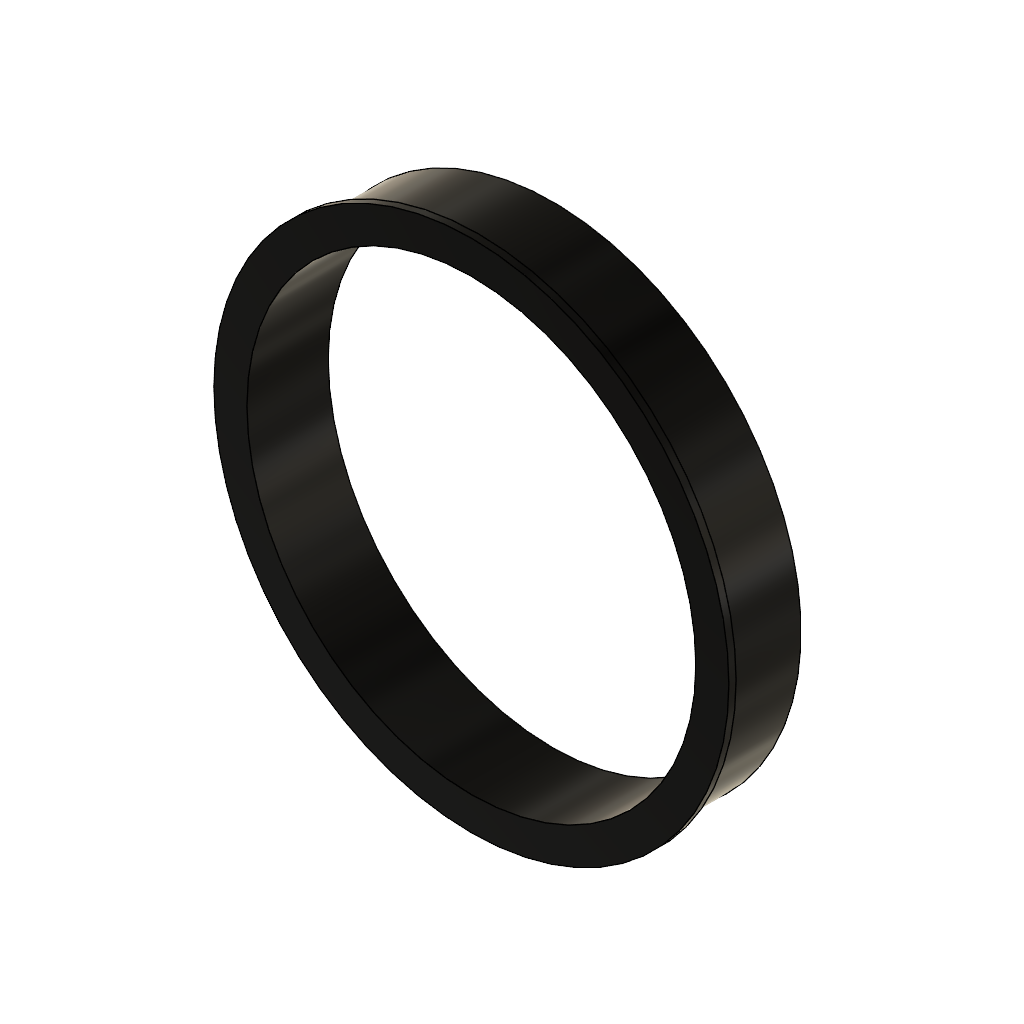
Rick Workshop cache difusant led (Autodesk Fusion 360 design; units mm, degrees)
Autodesk Fusion 360 part; units mm, degrees
(part 1 of 2)
sketch "Esquisse261" plane through (0, 0, 0) normal (0, 1, 0) x (1, 0, 0)
  spline S0 degree 5 poles (130.1631, -52) (130.1652, -52.1909) (130.1668, -52.5728) (130.1613, -53.1457) (130.1382, -53.9093) (130.0834, -54.8626) (130.0031, -55.814) (129.8983, -56.7629) (129.77, -57.7086) (129.6195, -58.6508) (129.4486, -59.5891) (129.2587, -60.5234) (129.0517, -61.4536) (128.8294, -62.3797) (128.5934, -63.3018) (128.3453, -64.2202) (128.0865, -65.1352) (127.8182, -66.0469) (127.5414, -66.9556) (127.2566, -67.8616) (126.9641, -68.7649) (126.6638, -69.6656) (126.3553, -70.5636) (126.0379, -71.4586) (125.7105, -72.3502) (125.372, -73.238) (125.0207, -74.1211) (124.6551, -74.9988) (124.2736, -75.8699) (123.8744, -76.7335) (123.4561, -77.5881) (123.0173, -78.4325) (122.5566, -79.2654) (122.0732, -80.0853) (121.5664, -80.891) (121.0359, -81.6814) (120.482, -82.4553) (119.9049, -83.212) (119.3056, -83.951) (118.685, -84.672) (118.0445, -85.3749) (117.3859, -86.0604) (116.7109, -86.7289) (116.0215, -87.3814) (115.3196, -88.0193) (114.6071, -88.6438) (113.8861, -89.2567) (113.1582, -89.8597) (112.4253, -90.4544) (111.6886, -91.0426) (110.9496, -91.6259) (110.2091, -92.2056) (109.4678, -92.7829) (108.7262, -93.3586) (107.9842, -93.9332) (107.2416, -94.5069) (106.4979, -95.0792) (105.7522, -95.6496) (105.0035, -96.2171) (104.2507, -96.7802) (103.4926, -97.3374) (102.7276, -97.8865) (101.9545, -98.4256) (101.1721, -98.9523) (100.3792, -99.4643) (99.5749, -99.9593) (98.7586, -100.4349) (97.9298, -100.8889) (97.0882, -101.3195) (96.234, -101.7248) (95.3676, -102.1035) (94.4896, -102.4546) (93.6008, -102.7773) (92.7022, -103.0714) (91.7948, -103.337) (90.8799, -103.5747) (89.9586, -103.7854) (89.032, -103.9704) (88.1014, -104.1309) (87.1676, -104.2689) (86.2317, -104.3859) (85.2943, -104.484) (84.3561, -104.565) (83.4176, -104.6306) (82.4793, -104.6826) (81.5414, -104.7223) (80.604, -104.751) (79.6674, -104.7697) (78.7314, -104.7791) (77.7963, -104.7795) (76.8619, -104.7712) (75.9281, -104.7539) (74.9951, -104.7273) (74.0628, -104.6909) (73.1313, -104.6439) (72.2006, -104.5856) (71.2709, -104.5153) (70.3424, -104.4321) (69.4152, -104.3354) (68.4896, -104.2249) (67.5659, -104.1002) (66.6441, -103.9612) (65.7246, -103.8083) (64.8075, -103.6417) (63.8927, -103.4623) (62.9801, -103.271) (62.0698, -103.0688) (61.1613, -102.8571) (60.2545, -102.6372) (59.3487, -102.4105) (58.4436, -102.1782) (57.5387, -101.9417) (56.6334, -101.702) (55.7272, -101.4598) (54.8197, -101.2157) (53.9106, -100.9697) (52.9998, -100.7218) (52.0871, -100.4712) (51.1726, -100.217) (50.2568, -99.9579) (49.3399, -99.6921) (48.4229, -99.4178) (47.5065, -99.1326) (46.5918, -98.8343) (45.6803, -98.5203) (44.7735, -98.1882) (43.8731, -97.8352) (42.981, -97.4592) (42.0992, -97.0577) (41.23, -96.6288) (40.3757, -96.1706) (39.5387, -95.6818) (38.7212, -95.1614) (37.9253, -94.6087) (37.1532, -94.0237) (36.4067, -93.4068) (35.6871, -92.7588) (34.9958, -92.081) (34.3335, -91.3748) (33.7005, -90.6421) (33.0966, -89.8852) (32.5213, -89.1063) (31.9736, -88.3077) (31.4525, -87.4919) (30.9562, -86.6612) (30.483, -85.8178) (30.031, -84.9638) (29.5982, -84.101) (29.1825, -83.2313) (28.782, -82.356) (28.3948, -81.4766) (28.0192, -80.5939) (27.6538, -79.7089) (27.2973, -78.8222) (26.9489, -77.934) (26.608, -77.0447) (26.2745, -76.1542) (25.9483, -75.2625) (25.6299, -74.3692) (25.32, -73.4741) (25.0194, -72.5768) (24.7292, -71.6769) (24.4507, -70.774) (24.1851, -69.8679) (23.9336, -68.9583) (23.6975, -68.0451) (23.4777, -67.1284) (23.2751, -66.2081) (23.0904, -65.2845) (22.924, -64.358) (22.7759, -63.4287) (22.646, -62.4973) (22.5338, -61.5642) (22.4386, -60.6297) (22.3595, -59.6944) (22.2954, -58.7586) (22.2449, -57.8226) (22.2069, -56.8867) (22.1799, -55.9511) (22.1626, -55.0159) (22.1541, -54.0811) (22.1532, -53.1467) (22.1592, -52.2127) (22.1717, -51.2789) (22.1905, -50.3453) (22.2159, -49.4117) (22.2483, -48.4781) (22.2886, -47.5444) (22.3379, -46.6107) (22.3975, -45.6771) (22.4689, -44.7437) (22.554, -43.811) (22.6545, -42.8792) (22.7721, -41.9489) (22.9085, -41.0207) (23.0653, -40.0954) (23.2439, -39.1738) (23.4453, -38.2567) (23.6703, -37.3448) (23.9194, -36.4392) (24.1926, -35.5404) (24.4896, -34.6492) (24.8097, -33.7661) (25.152, -32.8915) (25.5151, -32.0255) (25.8976, -31.168) (26.2975, -30.3189) (26.7131, -29.4776) (27.1425, -28.6436) (27.5836, -27.8161) (28.0346, -26.9944) (28.4938, -26.1774) (28.9597, -25.3644) (29.431, -24.5546) (29.9068, -23.7472) (30.3866, -22.9418) (30.8701, -22.1379) (31.3574, -21.3355) (31.8491, -20.5346) (32.346, -19.7357) (32.8492, -18.9394) (33.3602, -18.1466) (33.8807, -17.3584) (34.4122, -16.5763) (34.9567, -15.8018) (35.5159, -15.0367) (36.0914, -14.2827) (36.6849, -13.542) (37.2975, -12.8163) (37.9304, -12.1077) (38.5843, -11.4181) (39.2594, -10.7491) (39.956, -10.1023) (40.6736, -9.4789) (41.4116, -8.8797) (42.169, -8.3052) (42.9445, -7.7555) (43.7368, -7.2304) (44.5442, -6.7293) (45.3651, -6.251) (46.1977, -5.7942) (47.0404, -5.3571) (47.8915, -4.9379) (48.7494, -4.5345) (49.6129, -4.1448) (50.4806, -3.7666) (51.3515, -3.3979) (52.2248, -3.0368) (53.0998, -2.6815) (53.9761, -2.3308) (54.8533, -1.9835) (55.7316, -1.639) (56.6109, -1.297) (57.4916, -0.9574) (58.3739, -0.6209) (59.2585, -0.2882) (60.1459, 0.0395) (61.0367, 0.3607) (61.9314, 0.6738) (62.8306, 0.977) (63.7348, 1.2684) (64.6442, 1.5461) (65.5591, 1.8082) (66.4796, 2.053) (67.4056, 2.2787) (68.337, 2.484) (69.2733, 2.6676) (70.2143, 2.8286) (71.1593, 2.9663) (72.1077, 3.0802) (73.059, 3.1703) (74.0124, 3.2367) (74.9673, 3.2796) (75.9231, 3.2997) (76.8793, 3.2975) (77.8352, 3.2738) (78.7905, 3.2293) (79.7447, 3.1648) (80.6974, 3.0809) (81.6483, 2.9781) (82.597, 2.8567) (83.5432, 2.7169) (84.4865, 2.5588) (85.4264, 2.3819) (86.3625, 2.1859) (87.2942, 1.97) (88.2208, 1.7333) (89.1415, 1.475) (90.0554, 1.1938) (90.9615, 0.8888) (91.8587, 0.5587) (92.7458, 0.2027) (93.6216, -0.1801) (94.4847, -0.5904) (95.3341, -1.0285) (96.1684, -1.4944) (96.9867, -1.9878) (97.788, -2.5081) (98.5717, -3.0542) (99.3374, -3.6249) (100.085, -4.2184) (100.8147, -4.8327) (101.5271, -5.4657) (102.2229, -6.115) (102.9036, -6.778) (103.5705, -7.4522) (104.2254, -8.1349) (104.8703, -8.8236) (105.5075, -9.5157) (106.139, -10.2087) (106.7674, -10.9005) (107.3949, -11.589) (108.0235, -12.2724) (108.6553, -12.9494) (109.2917, -13.6191) (109.9341, -14.2808) (110.5832, -14.9344) (111.2394, -15.5802) (111.9027, -16.2191) (112.5726, -16.8523) (113.2481, -17.4814) (113.9279, -18.1084) (114.6104, -18.7353) (115.2936, -19.3645) (115.9755, -19.9983) (116.6539, -20.6388) (117.3265, -21.2882) (117.9909, -21.9484) (118.6449, -22.621) (119.2862, -23.3076) (119.9128, -24.0091) (120.5227, -24.7262) (121.1144, -25.4594) (121.6865, -26.2087) (122.2379, -26.974) (122.7679, -27.7548) (123.2761, -28.5504) (123.7624, -29.3599) (124.2271, -30.1824) (124.6706, -31.0169) (125.0937, -31.8624) (125.4973, -32.7177) (125.8824, -33.5819) (126.25, -34.4541) (126.601, -35.3335) (126.9365, -36.2195) (127.2571, -37.1115) (127.5635, -38.009) (127.856, -38.9117) (128.1347, -39.8193) (128.3994, -40.7318) (128.6498, -41.649) (128.8851, -42.5707) (129.1046, -43.497) (129.3072, -44.4277) (129.4916, -45.3626) (129.6566, -46.3017) (129.8008, -47.2445) (129.923, -48.1908) (130.0219, -49.1401) (130.0966, -50.0919) (130.1361, -50.8546) (130.1542, -51.4272) (130.161, -51.8091) (130.1631, -52) knots 0 0 0 0 0 0 0.00277778 0.00555556 0.00833333 0.01111111 0.01388889 0.01666667 0.01944444 0.02222222 0.025 0.02777778 0.03055556 0.03333333 0.03611111 0.03888889 0.04166667 0.04444444 0.04722222 0.05 0.05277778 0.05555556 0.05833333 0.06111111 0.06388889 0.06666667 0.06944444 0.07222222 0.075 0.07777778 0.08055556 0.08333333 0.08611111 0.08888889 0.09166667 0.09444444 0.09722222 0.1 0.10277778 0.10555556 0.10833333 0.11111111 0.11388889 0.11666667 0.11944444 0.12222222 0.125 0.12777778 0.13055556 0.13333333 0.13611111 0.13888889 0.14166667 0.14444444 0.14722222 0.15 0.15277778 0.15555556 0.15833333 0.16111111 0.16388889 0.16666667 0.16944444 0.17222222 0.175 0.17777778 0.18055556 0.18333333 0.18611111 0.18888889 0.19166667 0.19444444 0.19722222 0.2 0.20277778 0.20555556 0.20833333 0.21111111 0.21388889 0.21666667 0.21944444 0.22222222 0.225 0.22777778 0.23055556 0.23333333 0.23611111 0.23888889 0.24166667 0.24444444 0.24722222 0.25 0.25277778 0.25555556 0.25833333 0.26111111 0.26388889 0.26666667 0.26944444 0.27222222 0.275 0.27777778 0.28055556 0.28333333 0.28611111 0.28888889 0.29166667 0.29444444 0.29722222 0.3 0.30277778 0.30555556 0.30833333 0.31111111 0.31388889 0.31666667 0.31944444 0.32222222 0.325 0.32777778 0.33055556 0.33333333 0.33611111 0.33888889 0.34166667 0.34444444 0.34722222 0.35 0.35277778 0.35555556 0.35833333 0.36111111 0.36388889 0.36666667 0.36944444 0.37222222 0.375 0.37777778 0.38055556 0.38333333 0.38611111 0.38888889 0.39166667 0.39444444 0.39722222 0.4 0.40277778 0.40555556 0.40833333 0.41111111 0.41388889 0.41666667 0.41944444 0.42222222 0.425 0.42777778 0.43055556 0.43333333 0.43611111 0.43888889 0.44166667 0.44444444 0.44722222 0.45 0.45277778 0.45555556 0.45833333 0.46111111 0.46388889 0.46666667 0.46944444 0.47222222 0.475 0.47777778 0.48055556 0.48333333 0.48611111 0.48888889 0.49166667 0.49444444 0.49722222 0.5 0.50277778 0.50555556 0.50833333 0.51111111 0.51388889 0.51666667 0.51944444 0.52222222 0.525 0.52777778 0.53055556 0.53333333 0.53611111 0.53888889 0.54166667 0.54444444 0.54722222 0.55 0.55277778 0.55555556 0.55833333 0.56111111 0.56388889 0.56666667 0.56944444 0.57222222 0.575 0.57777778 0.58055556 0.58333333 0.58611111 0.58888889 0.59166667 0.59444444 0.59722222 0.6 0.60277778 0.60555556 0.60833333 0.61111111 0.61388889 0.61666667 0.61944444 0.62222222 0.625 0.62777778 0.63055556 0.63333333 0.63611111 0.63888889 0.64166667 0.64444444 0.64722222 0.65 0.65277778 0.65555556 0.65833333 0.66111111 0.66388889 0.66666667 0.66944444 0.67222222 0.675 0.67777778 0.68055556 0.68333333 0.68611111 0.68888889 0.69166667 0.69444444 0.69722222 0.7 0.70277778 0.70555556 0.70833333 0.71111111 0.71388889 0.71666667 0.71944444 0.72222222 0.725 0.72777778 0.73055556 0.73333333 0.73611111 0.73888889 0.74166667 0.74444444 0.74722222 0.75 0.75277778 0.75555556 0.75833333 0.76111111 0.76388889 0.76666667 0.76944444 0.77222222 0.775 0.77777778 0.78055556 0.78333333 0.78611111 0.78888889 0.79166667 0.79444444 0.79722222 0.8 0.80277778 0.80555556 0.80833333 0.81111111 0.81388889 0.81666667 0.81944444 0.82222222 0.825 0.82777778 0.83055556 0.83333333 0.83611111 0.83888889 0.84166667 0.84444444 0.84722222 0.85 0.85277778 0.85555556 0.85833333 0.86111111 0.86388889 0.86666667 0.86944444 0.87222222 0.875 0.87777778 0.88055556 0.88333333 0.88611111 0.88888889 0.89166667 0.89444444 0.89722222 0.9 0.90277778 0.90555556 0.90833333 0.91111111 0.91388889 0.91666667 0.91944444 0.92222222 0.925 0.92777778 0.93055556 0.93333333 0.93611111 0.93888889 0.94166667 0.94444444 0.94722222 0.95 0.95277778 0.95555556 0.95833333 0.96111111 0.96388889 0.96666667 0.96944444 0.97222222 0.975 0.97777778 0.98055556 0.98333333 0.98611111 0.98888889 0.99166667 0.99444444 0.99722222 1 1 1 1 1 1
  point P0 (129.8875, -56.802)
  point P1 (129.0306, -61.5271)
  point P2 (127.7867, -66.1442)
  point P3 (126.3133, -70.6765)
  point P4 (124.5955, -75.1268)
  point P5 (122.4683, -79.4059)
  point P6 (119.7816, -83.3564)
  point P7 (116.5566, -86.8701)
  point P8 (112.9923, -89.9923)
  point P9 (109.3181, -92.8988)
  point P10 (105.6287, -95.7423)
  point P11 (101.8445, -98.4961)
  point P12 (97.8206, -100.9389)
  point P13 (93.4921, -102.8066)
  point P14 (88.9288, -103.9831)
  point P15 (84.2691, -104.5679)
  point P16 (79.6166, -104.7681)
  point P17 (75, -104.725)
  point P18 (70.4125, -104.4354)
  point P19 (65.8613, -103.8284)
  point P20 (61.3608, -102.9022)
  point P21 (56.8858, -101.7685)
  point P22 (52.3625, -100.5463)
  point P23 (47.7461, -99.2052)
  point P24 (43.1291, -97.5163)
  point P25 (38.7674, -95.1804)
  point P26 (34.9651, -92.0349)
  point P27 (31.8931, -88.171)
  point P28 (29.4893, -83.8669)
  point P29 (27.5329, -79.4051)
  point P30 (25.8303, -74.9282)
  point P31 (24.3529, -70.434)
  point P32 (23.2113, -65.8767)
  point P33 (22.5048, -61.2563)
  point P34 (22.2007, -56.6193)
  point P35 (22.1631, -52)
  point P36 (22.2984, -47.3892)
  point P37 (22.6714, -42.7731)
  point P38 (23.4667, -38.1917)
  point P39 (24.8265, -33.7383)
  point P40 (26.7143, -29.484)
  point P41 (28.9376, -25.4059)
  point P42 (31.3132, -21.4102)
  point P43 (33.8238, -17.4491)
  point P44 (36.6248, -13.6248)
  point P45 (39.8971, -10.166)
  point P46 (43.6824, -7.2738)
  point P47 (47.8445, -4.9653)
  point P48 (52.1778, -3.0577)
  point P49 (56.5539, -1.3198)
  point P50 (60.9764, 0.3368)
  point P51 (65.5151, 1.7913)
  point P52 (70.2038, 2.8209)
  point P53 (75, 3.275)
  point P54 (79.8253, 3.1536)
  point P55 (84.6153, 2.5308)
  point P56 (89.3133, 1.4178)
  point P57 (93.8239, -0.2817)
  point P58 (98.0052, -2.6651)
  point P59 (101.7461, -5.6744)
  point P60 (105.0754, -9.0479)
  point P61 (108.1884, -12.4476)
  point P62 (111.3326, -15.6674)
  point P63 (114.6259, -18.75)
  point P64 (117.9578, -21.9206)
  point P65 (121.0637, -25.4051)
  point P66 (123.7115, -29.2854)
  point P67 (125.8397, -33.4958)
  point P68 (127.5313, -37.9243)
  point P69 (128.864, -42.5023)
  point P70 (129.7898, -47.2065)
extrude "Disque portail (usinage)" add sketch "Esquisse261" along normal blind 30 from surface at 25.75 makes body 1
sketch "Esquisse262" plane through (0, 0, 0) normal (0, 1, 0) x (1, 0, 0)
  line L0 (0, 70) -> (150, 70)
  line L1 (150, 70) -> (150, 0)
  line L2 (150, 0) -> (0, 0)
  line L3 (0, 0) -> (0, 70)
extrude "Socle - exterieur (usinage)" add sketch "Esquisse262" along normal blind 85 bodies 1
sketch "Esquisse263" plane through (0, 0, 0) normal (0, 1, 0) x (1, 0, 0)
  spline S0 degree 5 poles (130.1631, -52) (130.1652, -52.1909) (130.1668, -52.5728) (130.1613, -53.1457) (130.1382, -53.9093) (130.0834, -54.8626) (130.0031, -55.814) (129.8983, -56.7629) (129.77, -57.7086) (129.6195, -58.6508) (129.4486, -59.5891) (129.2587, -60.5234) (129.0517, -61.4536) (128.8294, -62.3797) (128.5934, -63.3018) (128.3453, -64.2202) (128.0865, -65.1352) (127.8182, -66.0469) (127.5414, -66.9556) (127.2566, -67.8616) (126.9641, -68.7649) (126.6638, -69.6656) (126.3553, -70.5636) (126.0379, -71.4586) (125.7105, -72.3502) (125.372, -73.238) (125.0207, -74.1211) (124.6551, -74.9988) (124.2736, -75.8699) (123.8744, -76.7335) (123.4561, -77.5881) (123.0173, -78.4325) (122.5566, -79.2654) (122.0732, -80.0853) (121.5664, -80.891) (121.0359, -81.6814) (120.482, -82.4553) (119.9049, -83.212) (119.3056, -83.951) (118.685, -84.672) (118.0445, -85.3749) (117.3859, -86.0604) (116.7109, -86.7289) (116.0215, -87.3814) (115.3196, -88.0193) (114.6071, -88.6438) (113.8861, -89.2567) (113.1582, -89.8597) (112.4253, -90.4544) (111.6886, -91.0426) (110.9496, -91.6259) (110.2091, -92.2056) (109.4678, -92.7829) (108.7262, -93.3586) (107.9842, -93.9332) (107.2416, -94.5069) (106.4979, -95.0792) (105.7522, -95.6496) (105.0035, -96.2171) (104.2507, -96.7802) (103.4926, -97.3374) (102.7276, -97.8865) (101.9545, -98.4256) (101.1721, -98.9523) (100.3792, -99.4643) (99.5749, -99.9593) (98.7586, -100.4349) (97.9298, -100.8889) (97.0882, -101.3195) (96.234, -101.7248) (95.3676, -102.1035) (94.4896, -102.4546) (93.6008, -102.7773) (92.7022, -103.0714) (91.7948, -103.337) (90.8799, -103.5747) (89.9586, -103.7854) (89.032, -103.9704) (88.1014, -104.1309) (87.1676, -104.2689) (86.2317, -104.3859) (85.2943, -104.484) (84.3561, -104.565) (83.4176, -104.6306) (82.4793, -104.6826) (81.5414, -104.7223) (80.604, -104.751) (79.6674, -104.7697) (78.7314, -104.7791) (77.7963, -104.7795) (76.8619, -104.7712) (75.9281, -104.7539) (74.9951, -104.7273) (74.0628, -104.6909) (73.1313, -104.6439) (72.2006, -104.5856) (71.2709, -104.5153) (70.3424, -104.4321) (69.4152, -104.3354) (68.4896, -104.2249) (67.5659, -104.1002) (66.6441, -103.9612) (65.7246, -103.8083) (64.8075, -103.6417) (63.8927, -103.4623) (62.9801, -103.271) (62.0698, -103.0688) (61.1613, -102.8571) (60.2545, -102.6372) (59.3487, -102.4105) (58.4436, -102.1782) (57.5387, -101.9417) (56.6334, -101.702) (55.7272, -101.4598) (54.8197, -101.2157) (53.9106, -100.9697) (52.9998, -100.7218) (52.0871, -100.4712) (51.1726, -100.217) (50.2568, -99.9579) (49.3399, -99.6921) (48.4229, -99.4178) (47.5065, -99.1326) (46.5918, -98.8343) (45.6803, -98.5203) (44.7735, -98.1882) (43.8731, -97.8352) (42.981, -97.4592) (42.0992, -97.0577) (41.23, -96.6288) (40.3757, -96.1706) (39.5387, -95.6818) (38.7212, -95.1614) (37.9253, -94.6087) (37.1532, -94.0237) (36.4067, -93.4068) (35.6871, -92.7588) (34.9958, -92.081) (34.3335, -91.3748) (33.7005, -90.6421) (33.0966, -89.8852) (32.5213, -89.1063) (31.9736, -88.3077) (31.4525, -87.4919) (30.9562, -86.6612) (30.483, -85.8178) (30.031, -84.9638) (29.5982, -84.101) (29.1825, -83.2313) (28.782, -82.356) (28.3948, -81.4766) (28.0192, -80.5939) (27.6538, -79.7089) (27.2973, -78.8222) (26.9489, -77.934) (26.608, -77.0447) (26.2745, -76.1542) (25.9483, -75.2625) (25.6299, -74.3692) (25.32, -73.4741) (25.0194, -72.5768) (24.7292, -71.6769) (24.4507, -70.774) (24.1851, -69.8679) (23.9336, -68.9583) (23.6975, -68.0451) (23.4777, -67.1284) (23.2751, -66.2081) (23.0904, -65.2845) (22.924, -64.358) (22.7759, -63.4287) (22.646, -62.4973) (22.5338, -61.5642) (22.4386, -60.6297) (22.3595, -59.6944) (22.2954, -58.7586) (22.2449, -57.8226) (22.2069, -56.8867) (22.1799, -55.9511) (22.1626, -55.0159) (22.1541, -54.0811) (22.1532, -53.1467) (22.1592, -52.2127) (22.1717, -51.2789) (22.1905, -50.3453) (22.2159, -49.4117) (22.2483, -48.4781) (22.2886, -47.5444) (22.3379, -46.6107) (22.3975, -45.6771) (22.4689, -44.7437) (22.554, -43.811) (22.6545, -42.8792) (22.7721, -41.9489) (22.9085, -41.0207) (23.0653, -40.0954) (23.2439, -39.1738) (23.4453, -38.2567) (23.6703, -37.3448) (23.9194, -36.4392) (24.1926, -35.5404) (24.4896, -34.6492) (24.8097, -33.7661) (25.152, -32.8915) (25.5151, -32.0255) (25.8976, -31.168) (26.2975, -30.3189) (26.7131, -29.4776) (27.1425, -28.6436) (27.5836, -27.8161) (28.0346, -26.9944) (28.4938, -26.1774) (28.9597, -25.3644) (29.431, -24.5546) (29.9068, -23.7472) (30.3866, -22.9418) (30.8701, -22.1379) (31.3574, -21.3355) (31.8491, -20.5346) (32.346, -19.7357) (32.8492, -18.9394) (33.3602, -18.1466) (33.8807, -17.3584) (34.4122, -16.5763) (34.9567, -15.8018) (35.5159, -15.0367) (36.0914, -14.2827) (36.6849, -13.542) (37.2975, -12.8163) (37.9304, -12.1077) (38.5843, -11.4181) (39.2594, -10.7491) (39.956, -10.1023) (40.6736, -9.4789) (41.4116, -8.8797) (42.169, -8.3052) (42.9445, -7.7555) (43.7368, -7.2304) (44.5442, -6.7293) (45.3651, -6.251) (46.1977, -5.7942) (47.0404, -5.3571) (47.8915, -4.9379) (48.7494, -4.5345) (49.6129, -4.1448) (50.4806, -3.7666) (51.3515, -3.3979) (52.2248, -3.0368) (53.0998, -2.6815) (53.9761, -2.3308) (54.8533, -1.9835) (55.7316, -1.639) (56.6109, -1.297) (57.4916, -0.9574) (58.3739, -0.6209) (59.2585, -0.2882) (60.1459, 0.0395) (61.0367, 0.3607) (61.9314, 0.6738) (62.8306, 0.977) (63.7348, 1.2684) (64.6442, 1.5461) (65.5591, 1.8082) (66.4796, 2.053) (67.4056, 2.2787) (68.337, 2.484) (69.2733, 2.6676) (70.2143, 2.8286) (71.1593, 2.9663) (72.1077, 3.0802) (73.059, 3.1703) (74.0124, 3.2367) (74.9673, 3.2796) (75.9231, 3.2997) (76.8793, 3.2975) (77.8352, 3.2738) (78.7905, 3.2293) (79.7447, 3.1648) (80.6974, 3.0809) (81.6483, 2.9781) (82.597, 2.8567) (83.5432, 2.7169) (84.4865, 2.5588) (85.4264, 2.3819) (86.3625, 2.1859) (87.2942, 1.97) (88.2208, 1.7333) (89.1415, 1.475) (90.0554, 1.1938) (90.9615, 0.8888) (91.8587, 0.5587) (92.7458, 0.2027) (93.6216, -0.1801) (94.4847, -0.5904) (95.3341, -1.0285) (96.1684, -1.4944) (96.9867, -1.9878) (97.788, -2.5081) (98.5717, -3.0542) (99.3374, -3.6249) (100.085, -4.2184) (100.8147, -4.8327) (101.5271, -5.4657) (102.2229, -6.115) (102.9036, -6.778) (103.5705, -7.4522) (104.2254, -8.1349) (104.8703, -8.8236) (105.5075, -9.5157) (106.139, -10.2087) (106.7674, -10.9005) (107.3949, -11.589) (108.0235, -12.2724) (108.6553, -12.9494) (109.2917, -13.6191) (109.9341, -14.2808) (110.5832, -14.9344) (111.2394, -15.5802) (111.9027, -16.2191) (112.5726, -16.8523) (113.2481, -17.4814) (113.9279, -18.1084) (114.6104, -18.7353) (115.2936, -19.3645) (115.9755, -19.9983) (116.6539, -20.6388) (117.3265, -21.2882) (117.9909, -21.9484) (118.6449, -22.621) (119.2862, -23.3076) (119.9128, -24.0091) (120.5227, -24.7262) (121.1144, -25.4594) (121.6865, -26.2087) (122.2379, -26.974) (122.7679, -27.7548) (123.2761, -28.5504) (123.7624, -29.3599) (124.2271, -30.1824) (124.6706, -31.0169) (125.0937, -31.8624) (125.4973, -32.7177) (125.8824, -33.5819) (126.25, -34.4541) (126.601, -35.3335) (126.9365, -36.2195) (127.2571, -37.1115) (127.5635, -38.009) (127.856, -38.9117) (128.1347, -39.8193) (128.3994, -40.7318) (128.6498, -41.649) (128.8851, -42.5707) (129.1046, -43.497) (129.3072, -44.4277) (129.4916, -45.3626) (129.6566, -46.3017) (129.8008, -47.2445) (129.923, -48.1908) (130.0219, -49.1401) (130.0966, -50.0919) (130.1361, -50.8546) (130.1542, -51.4272) (130.161, -51.8091) (130.1631, -52) knots 0 0 0 0 0 0 0.00277778 0.00555556 0.00833333 0.01111111 0.01388889 0.01666667 0.01944444 0.02222222 0.025 0.02777778 0.03055556 0.03333333 0.03611111 0.03888889 0.04166667 0.04444444 0.04722222 0.05 0.05277778 0.05555556 0.05833333 0.06111111 0.06388889 0.06666667 0.06944444 0.07222222 0.075 0.07777778 0.08055556 0.08333333 0.08611111 0.08888889 0.09166667 0.09444444 0.09722222 0.1 0.10277778 0.10555556 0.10833333 0.11111111 0.11388889 0.11666667 0.11944444 0.12222222 0.125 0.12777778 0.13055556 0.13333333 0.13611111 0.13888889 0.14166667 0.14444444 0.14722222 0.15 0.15277778 0.15555556 0.15833333 0.16111111 0.16388889 0.16666667 0.16944444 0.17222222 0.175 0.17777778 0.18055556 0.18333333 0.18611111 0.18888889 0.19166667 0.19444444 0.19722222 0.2 0.20277778 0.20555556 0.20833333 0.21111111 0.21388889 0.21666667 0.21944444 0.22222222 0.225 0.22777778 0.23055556 0.23333333 0.23611111 0.23888889 0.24166667 0.24444444 0.24722222 0.25 0.25277778 0.25555556 0.25833333 0.26111111 0.26388889 0.26666667 0.26944444 0.27222222 0.275 0.27777778 0.28055556 0.28333333 0.28611111 0.28888889 0.29166667 0.29444444 0.29722222 0.3 0.30277778 0.30555556 0.30833333 0.31111111 0.31388889 0.31666667 0.31944444 0.32222222 0.325 0.32777778 0.33055556 0.33333333 0.33611111 0.33888889 0.34166667 0.34444444 0.34722222 0.35 0.35277778 0.35555556 0.35833333 0.36111111 0.36388889 0.36666667 0.36944444 0.37222222 0.375 0.37777778 0.38055556 0.38333333 0.38611111 0.38888889 0.39166667 0.39444444 0.39722222 0.4 0.40277778 0.40555556 0.40833333 0.41111111 0.41388889 0.41666667 0.41944444 0.42222222 0.425 0.42777778 0.43055556 0.43333333 0.43611111 0.43888889 0.44166667 0.44444444 0.44722222 0.45 0.45277778 0.45555556 0.45833333 0.46111111 0.46388889 0.46666667 0.46944444 0.47222222 0.475 0.47777778 0.48055556 0.48333333 0.48611111 0.48888889 0.49166667 0.49444444 0.49722222 0.5 0.50277778 0.50555556 0.50833333 0.51111111 0.51388889 0.51666667 0.51944444 0.52222222 0.525 0.52777778 0.53055556 0.53333333 0.53611111 0.53888889 0.54166667 0.54444444 0.54722222 0.55 0.55277778 0.55555556 0.55833333 0.56111111 0.56388889 0.56666667 0.56944444 0.57222222 0.575 0.57777778 0.58055556 0.58333333 0.58611111 0.58888889 0.59166667 0.59444444 0.59722222 0.6 0.60277778 0.60555556 0.60833333 0.61111111 0.61388889 0.61666667 0.61944444 0.62222222 0.625 0.62777778 0.63055556 0.63333333 0.63611111 0.63888889 0.64166667 0.64444444 0.64722222 0.65 0.65277778 0.65555556 0.65833333 0.66111111 0.66388889 0.66666667 0.66944444 0.67222222 0.675 0.67777778 0.68055556 0.68333333 0.68611111 0.68888889 0.69166667 0.69444444 0.69722222 0.7 0.70277778 0.70555556 0.70833333 0.71111111 0.71388889 0.71666667 0.71944444 0.72222222 0.725 0.72777778 0.73055556 0.73333333 0.73611111 0.73888889 0.74166667 0.74444444 0.74722222 0.75 0.75277778 0.75555556 0.75833333 0.76111111 0.76388889 0.76666667 0.76944444 0.77222222 0.775 0.77777778 0.78055556 0.78333333 0.78611111 0.78888889 0.79166667 0.79444444 0.79722222 0.8 0.80277778 0.80555556 0.80833333 0.81111111 0.81388889 0.81666667 0.81944444 0.82222222 0.825 0.82777778 0.83055556 0.83333333 0.83611111 0.83888889 0.84166667 0.84444444 0.84722222 0.85 0.85277778 0.85555556 0.85833333 0.86111111 0.86388889 0.86666667 0.86944444 0.87222222 0.875 0.87777778 0.88055556 0.88333333 0.88611111 0.88888889 0.89166667 0.89444444 0.89722222 0.9 0.90277778 0.90555556 0.90833333 0.91111111 0.91388889 0.91666667 0.91944444 0.92222222 0.925 0.92777778 0.93055556 0.93333333 0.93611111 0.93888889 0.94166667 0.94444444 0.94722222 0.95 0.95277778 0.95555556 0.95833333 0.96111111 0.96388889 0.96666667 0.96944444 0.97222222 0.975 0.97777778 0.98055556 0.98333333 0.98611111 0.98888889 0.99166667 0.99444444 0.99722222 1 1 1 1 1 1
  spline S1 degree 5 poles (123.1631, -52) (123.1652, -52.1666) (123.167, -52.4997) (123.1624, -52.9994) (123.1419, -53.6656) (123.0924, -54.4971) (123.0197, -55.3268) (122.9244, -56.1541) (122.8078, -56.9784) (122.6713, -57.7994) (122.5162, -58.6168) (122.3444, -59.4305) (122.1576, -60.2403) (121.9575, -61.0465) (121.7457, -61.8491) (121.5239, -62.6484) (121.2935, -63.4447) (121.0557, -64.2383) (120.8113, -65.0295) (120.561, -65.8186) (120.305, -66.6056) (120.0432, -67.3906) (119.7752, -68.1736) (119.5004, -68.9543) (119.2175, -69.7325) (118.9255, -70.5075) (118.6227, -71.2788) (118.3076, -72.0454) (117.9784, -72.8065) (117.6337, -73.5608) (117.2717, -74.3073) (116.891, -75.0446) (116.4903, -75.7713) (116.0688, -76.4862) (115.6257, -77.188) (115.1609, -77.8756) (114.6743, -78.548) (114.1664, -79.2042) (113.638, -79.8439) (113.0901, -80.4668) (112.5241, -81.073) (111.9416, -81.6629) (111.3444, -82.2371) (110.7343, -82.7967) (110.1134, -83.3429) (109.4834, -83.8772) (108.8464, -84.4013) (108.2041, -84.9169) (107.558, -85.4257) (106.9097, -85.9295) (106.2604, -86.4299) (105.6109, -86.9284) (104.9621, -87.4261) (104.3142, -87.9239) (103.6674, -88.4223) (103.0212, -88.9214) (102.3753, -89.4209) (101.7287, -89.9203) (101.0804, -90.4184) (100.4293, -90.914) (99.7739, -91.4054) (99.113, -91.8906) (98.4451, -92.3676) (97.7689, -92.834) (97.0833, -93.2877) (96.3873, -93.7262) (95.6801, -94.1472) (94.9613, -94.5486) (94.2307, -94.9285) (93.4883, -95.2851) (92.7345, -95.617) (91.9699, -95.9233) (91.1952, -96.2031) (90.4115, -96.4564) (89.6197, -96.6831) (88.821, -96.8839) (88.0167, -97.0597) (87.2077, -97.2118) (86.3953, -97.3415) (85.5803, -97.4507) (84.7636, -97.541) (83.946, -97.6145) (83.128, -97.6729) (82.31, -97.7181) (81.4926, -97.7516) (80.6758, -97.7751) (79.8598, -97.7897) (79.0447, -97.7964) (78.2305, -97.7959) (77.4172, -97.7887) (76.6046, -97.7748) (75.7929, -97.7541) (74.9819, -97.7263) (74.1716, -97.6907) (73.3619, -97.6467) (72.5531, -97.5936) (71.7452, -97.5305) (70.9382, -97.4567) (70.1325, -97.3715) (69.3281, -97.2746) (68.5253, -97.1656) (67.7242, -97.0445) (66.925, -96.9115) (66.1277, -96.7671) (65.3324, -96.6119) (64.539, -96.4469) (63.7472, -96.2733) (62.9567, -96.0923) (62.1673, -95.9052) (61.3784, -95.7135) (60.5895, -95.5184) (59.8001, -95.3212) (59.0096, -95.1228) (58.2176, -94.9242) (57.4236, -94.7256) (56.6273, -94.5271) (55.8285, -94.3286) (55.0272, -94.1293) (54.2235, -93.9283) (53.4175, -93.7241) (52.6099, -93.515) (51.8012, -93.299) (50.9923, -93.074) (50.1843, -92.8374) (49.3785, -92.5869) (48.5762, -92.3199) (47.7791, -92.0339) (46.9891, -91.7265) (46.2081, -91.3954) (45.4384, -91.0386) (44.682, -90.6544) (43.9413, -90.2412) (43.2186, -89.798) (42.5161, -89.3242) (41.8356, -88.8198) (41.1791, -88.2852) (40.5481, -87.721) (39.9437, -87.1286) (39.3667, -86.5094) (38.8174, -85.8654) (38.2957, -85.1987) (37.801, -84.5115) (37.3323, -83.8062) (36.8885, -83.0852) (36.4679, -82.3507) (36.0687, -81.6049) (35.6891, -80.8497) (35.327, -80.0871) (34.9804, -79.3187) (34.6472, -78.5459) (34.3256, -77.7699) (34.014, -76.9918) (33.7107, -76.2123) (33.4147, -75.432) (33.1249, -74.6512) (32.8408, -73.8702) (32.5621, -73.0889) (32.2889, -72.3072) (32.0216, -71.5248) (31.7606, -70.7415) (31.5071, -69.9568) (31.2619, -69.1703) (31.0263, -68.3816) (30.8016, -67.5904) (30.5889, -66.7964) (30.3894, -65.9996) (30.2043, -65.1997) (30.0342, -64.397) (29.88, -63.5915) (29.742, -62.7836) (29.6203, -61.9735) (29.5147, -61.1616) (29.4248, -60.3484) (29.3498, -59.5343) (29.2889, -58.7196) (29.2409, -57.9048) (29.2045, -57.09) (29.1785, -56.2755) (29.1614, -55.4615) (29.152, -54.648) (29.1492, -53.835) (29.1519, -53.0225) (29.1594, -52.2104) (29.1712, -51.3986) (29.1871, -50.5868) (29.2075, -49.7751) (29.2327, -48.9632) (29.2636, -48.1512) (29.3012, -47.3389) (29.3471, -46.5266) (29.4027, -45.7142) (29.4697, -44.9022) (29.55, -44.0908) (29.6454, -43.2805) (29.7574, -42.4719) (29.8878, -41.6658) (30.0378, -40.8628) (30.2087, -40.0637) (30.4012, -39.2694) (30.6157, -38.4807) (30.8522, -37.6982) (31.1106, -36.9227) (31.3902, -36.1546) (31.6899, -35.3942) (32.0086, -34.6417) (32.3445, -33.897) (32.696, -33.1597) (33.0612, -32.4295) (33.4381, -31.7057) (33.8249, -30.9874) (34.2197, -30.2739) (34.6208, -29.5641) (35.0266, -28.8573) (35.436, -28.1524) (35.8481, -27.449) (36.2622, -26.7463) (36.6782, -26.044) (37.0962, -25.342) (37.5169, -24.6404) (37.941, -23.9395) (38.3697, -23.24) (38.8046, -22.5428) (39.2473, -21.849) (39.6995, -21.16) (40.1631, -20.4772) (40.6399, -19.8023) (41.1315, -19.1373) (41.6396, -18.4839) (42.1655, -17.8442) (42.7101, -17.22) (43.2744, -16.6132) (43.8585, -16.0254) (44.4627, -15.4582) (45.0866, -14.9127) (45.7296, -14.3898) (46.3906, -13.8899) (47.0685, -13.4132) (47.7617, -12.9594) (48.4688, -12.5277) (49.1882, -12.1171) (49.918, -11.7261) (50.6567, -11.3531) (51.4026, -10.9961) (52.1544, -10.653) (52.9105, -10.3217) (53.67, -10) (54.4317, -9.6858) (55.1948, -9.3772) (55.9588, -9.0725) (56.7232, -8.7704) (57.4878, -8.4697) (58.2526, -8.1697) (59.0177, -7.8702) (59.7834, -7.5712) (60.5501, -7.2733) (61.3183, -6.9772) (62.0887, -6.6842) (62.8619, -6.3956) (63.6384, -6.1132) (64.4189, -5.8386) (65.2038, -5.5739) (65.9935, -5.3208) (66.7884, -5.0813) (67.5885, -4.8571) (68.3938, -4.6498) (69.2042, -4.4609) (70.0193, -4.2916) (70.8388, -4.1428) (71.6622, -4.0151) (72.4889, -3.9091) (73.3183, -3.8247) (74.1498, -3.762) (74.9828, -3.7205) (75.8167, -3.6997) (76.651, -3.6991) (77.4851, -3.7178) (78.3187, -3.7552) (79.1513, -3.8105) (79.9827, -3.883) (80.8124, -3.9724) (81.6402, -4.0781) (82.4658, -4.2002) (83.2888, -4.3386) (84.1088, -4.4935) (84.9254, -4.6655) (85.738, -4.8554) (86.5459, -5.0638) (87.3485, -5.2919) (88.1448, -5.5408) (88.934, -5.8114) (89.7148, -6.105) (90.4861, -6.4225) (91.2468, -6.7647) (91.9955, -7.1324) (92.7311, -7.5257) (93.4524, -7.9448) (94.1585, -8.3893) (94.8483, -8.8585) (95.5213, -9.3516) (96.1772, -9.8672) (96.8158, -10.4035) (97.4375, -10.9587) (98.0428, -11.5306) (98.6326, -12.1168) (99.2081, -12.7151) (99.771, -13.3227) (100.323, -13.9373) (100.8662, -14.5562) (101.4027, -15.177) (101.9349, -15.7973) (102.4651, -16.4148) (102.9958, -17.0277) (103.5291, -17.6341) (104.067, -18.2325) (104.6112, -18.8221) (105.1629, -19.4021) (105.7229, -19.9724) (106.2918, -20.5332) (106.8693, -21.0853) (107.4551, -21.6301) (108.0481, -22.1691) (108.647, -22.7043) (109.2501, -23.2379) (109.8556, -23.7724) (110.4613, -24.3099) (111.065, -24.8528) (111.6646, -25.4033) (112.2577, -25.9634) (112.8421, -26.5348) (113.4156, -27.1189) (113.9762, -27.7168) (114.522, -28.3292) (115.0515, -28.9568) (115.5632, -29.5995) (116.0561, -30.2572) (116.5296, -30.9294) (116.9832, -31.6156) (117.417, -32.3148) (117.831, -33.0261) (118.2258, -33.7486) (118.6023, -34.4813) (118.9611, -35.223) (119.3035, -35.9729) (119.6304, -36.7301) (119.9428, -37.4938) (120.2416, -38.2634) (120.5276, -39.0383) (120.8014, -39.8182) (121.0634, -40.6028) (121.3137, -41.3918) (121.552, -42.1851) (121.7781, -42.9827) (121.9912, -43.7844) (122.1905, -44.5903) (122.375, -45.4003) (122.5434, -46.2142) (122.6945, -47.032) (122.827, -47.8535) (122.9396, -48.6782) (123.031, -49.5058) (123.1003, -50.3356) (123.1373, -51.0009) (123.1544, -51.5004) (123.161, -51.8334) (123.1631, -52) knots 0 0 0 0 0 0 0.00277778 0.00555556 0.00833333 0.01111111 0.01388889 0.01666667 0.01944444 0.02222222 0.025 0.02777778 0.03055556 0.03333333 0.03611111 0.03888889 0.04166667 0.04444444 0.04722222 0.05 0.05277778 0.05555556 0.05833333 0.06111111 0.06388889 0.06666667 0.06944444 0.07222222 0.075 0.07777778 0.08055556 0.08333333 0.08611111 0.08888889 0.09166667 0.09444444 0.09722222 0.1 0.10277778 0.10555556 0.10833333 0.11111111 0.11388889 0.11666667 0.11944444 0.12222222 0.125 0.12777778 0.13055556 0.13333333 0.13611111 0.13888889 0.14166667 0.14444444 0.14722222 0.15 0.15277778 0.15555556 0.15833333 0.16111111 0.16388889 0.16666667 0.16944444 0.17222222 0.175 0.17777778 0.18055556 0.18333333 0.18611111 0.18888889 0.19166667 0.19444444 0.19722222 0.2 0.20277778 0.20555556 0.20833333 0.21111111 0.21388889 0.21666667 0.21944444 0.22222222 0.225 0.22777778 0.23055556 0.23333333 0.23611111 0.23888889 0.24166667 0.24444444 0.24722222 0.25 0.25277778 0.25555556 0.25833333 0.26111111 0.26388889 0.26666667 0.26944444 0.27222222 0.275 0.27777778 0.28055556 0.28333333 0.28611111 0.28888889 0.29166667 0.29444444 0.29722222 0.3 0.30277778 0.30555556 0.30833333 0.31111111 0.31388889 0.31666667 0.31944444 0.32222222 0.325 0.32777778 0.33055556 0.33333333 0.33611111 0.33888889 0.34166667 0.34444444 0.34722222 0.35 0.35277778 0.35555556 0.35833333 0.36111111 0.36388889 0.36666667 0.36944444 0.37222222 0.375 0.37777778 0.38055556 0.38333333 0.38611111 0.38888889 0.39166667 0.39444444 0.39722222 0.4 0.40277778 0.40555556 0.40833333 0.41111111 0.41388889 0.41666667 0.41944444 0.42222222 0.425 0.42777778 0.43055556 0.43333333 0.43611111 0.43888889 0.44166667 0.44444444 0.44722222 0.45 0.45277778 0.45555556 0.45833333 0.46111111 0.46388889 0.46666667 0.46944444 0.47222222 0.475 0.47777778 0.48055556 0.48333333 0.48611111 0.48888889 0.49166667 0.49444444 0.49722222 0.5 0.50277778 0.50555556 0.50833333 0.51111111 0.51388889 0.51666667 0.51944444 0.52222222 0.525 0.52777778 0.53055556 0.53333333 0.53611111 0.53888889 0.54166667 0.54444444 0.54722222 0.55 0.55277778 0.55555556 0.55833333 0.56111111 0.56388889 0.56666667 0.56944444 0.57222222 0.575 0.57777778 0.58055556 0.58333333 0.58611111 0.58888889 0.59166667 0.59444444 0.59722222 0.6 0.60277778 0.60555556 0.60833333 0.61111111 0.61388889 0.61666667 0.61944444 0.62222222 0.625 0.62777778 0.63055556 0.63333333 0.63611111 0.63888889 0.64166667 0.64444444 0.64722222 0.65 0.65277778 0.65555556 0.65833333 0.66111111 0.66388889 0.66666667 0.66944444 0.67222222 0.675 0.67777778 0.68055556 0.68333333 0.68611111 0.68888889 0.69166667 0.69444444 0.69722222 0.7 0.70277778 0.70555556 0.70833333 0.71111111 0.71388889 0.71666667 0.71944444 0.72222222 0.725 0.72777778 0.73055556 0.73333333 0.73611111 0.73888889 0.74166667 0.74444444 0.74722222 0.75 0.75277778 0.75555556 0.75833333 0.76111111 0.76388889 0.76666667 0.76944444 0.77222222 0.775 0.77777778 0.78055556 0.78333333 0.78611111 0.78888889 0.79166667 0.79444444 0.79722222 0.8 0.80277778 0.80555556 0.80833333 0.81111111 0.81388889 0.81666667 0.81944444 0.82222222 0.825 0.82777778 0.83055556 0.83333333 0.83611111 0.83888889 0.84166667 0.84444444 0.84722222 0.85 0.85277778 0.85555556 0.85833333 0.86111111 0.86388889 0.86666667 0.86944444 0.87222222 0.875 0.87777778 0.88055556 0.88333333 0.88611111 0.88888889 0.89166667 0.89444444 0.89722222 0.9 0.90277778 0.90555556 0.90833333 0.91111111 0.91388889 0.91666667 0.91944444 0.92222222 0.925 0.92777778 0.93055556 0.93333333 0.93611111 0.93888889 0.94166667 0.94444444 0.94722222 0.95 0.95277778 0.95555556 0.95833333 0.96111111 0.96388889 0.96666667 0.96944444 0.97222222 0.975 0.97777778 0.98055556 0.98333333 0.98611111 0.98888889 0.99166667 0.99444444 0.99722222 1 1 1 1 1 1
  point P0 (129.8875, -56.802)
  point P1 (129.0306, -61.5271)
  point P2 (127.7867, -66.1442)
  point P3 (126.3133, -70.6765)
  point P4 (124.5955, -75.1268)
  point P5 (122.4683, -79.4059)
  point P6 (119.7816, -83.3564)
  point P7 (116.5566, -86.8701)
  point P8 (112.9923, -89.9923)
  point P9 (109.3181, -92.8988)
  point P10 (105.6287, -95.7423)
  point P11 (101.8445, -98.4961)
  point P12 (97.8206, -100.9389)
  point P13 (93.4921, -102.8066)
  point P14 (88.9288, -103.9831)
  point P15 (84.2691, -104.5679)
  point P16 (79.6166, -104.7681)
  point P17 (75, -104.725)
  point P18 (70.4125, -104.4354)
  point P19 (65.8613, -103.8284)
  point P20 (61.3608, -102.9022)
  point P21 (56.8858, -101.7685)
  point P22 (52.3625, -100.5463)
  point P23 (47.7461, -99.2052)
  point P24 (43.1291, -97.5163)
  point P25 (38.7674, -95.1804)
  point P26 (34.9651, -92.0349)
  point P27 (31.8931, -88.171)
  point P28 (29.4893, -83.8669)
  point P29 (27.5329, -79.4051)
  point P30 (25.8303, -74.9282)
  point P31 (24.3529, -70.434)
  point P32 (23.2113, -65.8767)
  point P33 (22.5048, -61.2563)
  point P34 (22.2007, -56.6193)
  point P35 (22.1631, -52)
  point P36 (22.2984, -47.3892)
  point P37 (22.6714, -42.7731)
  point P38 (23.4667, -38.1917)
  point P39 (24.8265, -33.7383)
  point P40 (26.7143, -29.484)
  point P41 (28.9376, -25.4059)
  point P42 (31.3132, -21.4102)
  point P43 (33.8238, -17.4491)
  point P44 (36.6248, -13.6248)
  point P45 (39.8971, -10.166)
  point P46 (43.6824, -7.2738)
  point P47 (47.8445, -4.9653)
  point P48 (52.1778, -3.0577)
  point P49 (56.5539, -1.3198)
  point P50 (60.9764, 0.3368)
  point P51 (65.5151, 1.7913)
  point P52 (70.2038, 2.8209)
  point P53 (75, 3.275)
  point P54 (79.8253, 3.1536)
  point P55 (84.6153, 2.5308)
  point P56 (89.3133, 1.4178)
  point P57 (93.8239, -0.2817)
  point P58 (98.0052, -2.6651)
  point P59 (101.7461, -5.6744)
  point P60 (105.0754, -9.0479)
  point P61 (108.1884, -12.4476)
  point P62 (111.3326, -15.6674)
  point P63 (114.6259, -18.75)
  point P64 (117.9578, -21.9206)
  point P65 (121.0637, -25.4051)
  point P66 (123.7115, -29.2854)
  point P67 (125.8397, -33.4958)
  point P68 (127.5313, -37.9243)
  point P69 (128.864, -42.5023)
  point P70 (129.7898, -47.2065)
  point P71 (122.9141, -56.1919)
  point P72 (122.137, -60.3115)
  point P73 (121.0252, -64.3324)
  point P74 (119.7355, -68.2824)
  point P75 (118.2513, -72.1684)
  point P76 (116.4062, -75.9059)
  point P77 (114.0475, -79.3414)
  point P78 (111.1943, -82.3706)
  point P79 (108.0426, -85.0426)
  point P80 (104.8186, -87.5365)
  point P81 (101.6136, -90.0082)
  point P82 (98.3445, -92.4339)
  point P83 (94.8623, -94.5948)
  point P84 (91.098, -96.2288)
  point P85 (87.1171, -97.2217)
  point P86 (83.0536, -97.6742)
  point P87 (79.0065, -97.7947)
  point P88 (75, -97.725)
  point P89 (71.0226, -97.4621)
  point P90 (67.0768, -96.9347)
  point P91 (63.1725, -96.1407)
  point P92 (59.2799, -95.1906)
  point P93 (55.3208, -94.2022)
  point P94 (51.2461, -93.143)
  point P95 (47.1442, -91.7822)
  point P96 (43.2669, -89.8181)
  point P97 (39.9148, -87.0852)
  point P98 (37.2554, -83.6715)
  point P99 (35.2234, -79.8519)
  point P100 (33.5951, -75.9051)
  point P101 (32.1745, -71.9699)
  point P102 (30.9308, -68.0399)
  point P103 (29.9728, -64.065)
  point P104 (29.3984, -60.0408)
  point P105 (29.1741, -56.0092)
  point P106 (29.1631, -52)
  point P107 (29.2718, -47.9993)
  point P108 (29.565, -43.9886)
  point P109 (30.2282, -40.0034)
  point P110 (31.4044, -36.1325)
  point P111 (33.0584, -32.4423)
  point P112 (34.9998, -28.9059)
  point P113 (37.0472, -25.4252)
  point P114 (39.1861, -21.9486)
  point P115 (41.5745, -18.5745)
  point P116 (44.3966, -15.5283)
  point P117 (47.6974, -13.0079)
  point P118 (51.3445, -11.0275)
  point P119 (55.1362, -9.4018)
  point P120 (58.9481, -7.8977)
  point P121 (62.7881, -6.4246)
  point P122 (66.7307, -5.1023)
  point P123 (70.8139, -4.1524)
  point P124 (75, -3.725)
  point P125 (79.2152, -3.8198)
  point P126 (83.3997, -4.3628)
  point P127 (87.5015, -5.3437)
  point P128 (91.4298, -6.8595)
  point P129 (95.0469, -9.0093)
  point P130 (98.2461, -11.7366)
  point P131 (101.0604, -14.7819)
  point P132 (103.6889, -17.8099)
  point P133 (106.3828, -20.6172)
  point P134 (109.2635, -23.2495)
  point P135 (112.2237, -25.9357)
  point P136 (115.0015, -28.9051)
  point P137 (117.3674, -32.2438)
  point P138 (119.2619, -35.89)
  point P139 (120.7698, -39.736)
  point P140 (121.9704, -43.7179)
  point P141 (122.8164, -47.8166)
extrude "Jonc du portail (usinage)" add sketch "Esquisse263" along normal blind 3.5 from surface at 22.25 bodies 1
ref_plane "Plan de construction30" through (0, 25.75, 0) normal (0, 1, 0) x (0, 0, 1)